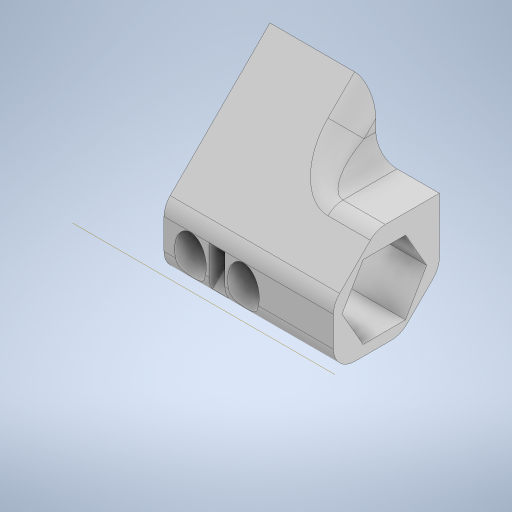
# Autodesk Inventor part: 2lickportv7
Saved by Autodesk Inventor 2024 (Build 280153000, 153)
## iProperties
Created: 2024-10-07
Part Number: 2lickportv7
Material: Generic
Document SubType Name: Modeling
Designer: xxred
Density: 1 g/cm^3
Appearance: Default
Author: xxred
Autodesk Inventor part; units mm, degrees
ref_plane "YZ Plane" through (0, 0, 0) normal (1, 0, 0) x (0, 1, 0)
ref_plane "XZ Plane" through (0, 0, 0) normal (0, 1, 0) x (-1, 0, 0)
ref_plane "XY Plane" through (0, 0, 0) normal (0, 0, 1) x (1, 0, 0)
sketch "Sketch2" plane through (0, 0, 0) normal (0, 1, 0) x (-1, 0, 0)
  line L0 (0, 0) -> (10, 0)
  line L1 (10, 0) -> (10, -10)
  line L2 (10, -10) -> (0, -10)
  line L3 (0, -10) -> (0, 0)
  dimension "d0" = 10
  dimension "d1" = 10
  constraints: 8 end point, 2 parallel, 1 horizontal, 1 perpendicular
  measures "d0" distance of L1.end L2.end
  measures "d1" distance of L0.end L1.end
extrude "Extrusion1" add sketch "Sketch2" along normal blind 20
ref_plane "Work Plane1" through (-10, 0, 0) normal (0, -0.7071068, 0.7071068) x (1, 0, 0)
sketch "Sketch3" plane through (-10, 0, 0) normal (0, -0.7071068, 0.7071068) x (1, 0, 0)
  circle A0 centre (2.5, 1.9025) radius 1.5
  circle A1 centre (7.5, 1.9025) radius 1.5
  line L0 (0, -7.0711) -> (0, 7.0711) projected
  line L1 (10, 0) -> (10, 14.1421) projected
  line L2 (0, 4.0177) -> (10, 4.0177)
  line L3 (10, 4.0177) -> (10, 14.1421)
  line L4 (10, 14.1421) -> (0, 14.1421)
  line L5 (0, 14.1421) -> (0, 4.0177)
  line L6 (2.5, 1.9025) -> (2.5, -0.2127)
  line L7 (2.5, 1.9025) -> (2.5, 4.0177)
  line L8 (4.25, 0.4025) -> (5.75, 0.4025)
  line L9 (5.75, 0.4025) -> (5.75, 3.4025)
  line L10 (5.75, 3.4025) -> (4.25, 3.4025)
  line L11 (4.25, 3.4025) -> (4.25, 0.4025)
  line L12 (7.5, 1.9025) -> (5.75, 1.9025)
  line L13 (4.25, 1.9025) -> (2.5, 1.9025)
  point P0 (10, 7.0711)
  dimension "d5" = 3
  dimension "d6" = 3
  dimension "d7" = 5
  dimension "d10" = 2.5
  dimension "d11" = 2.5
  dimension "d17" = 1.5
  dimension "d18" = 3
  constraints: 24 end point, 5 equal length, 3 perpendicular, 2 centre point, 2 collinear, 2 horizontal, 2 midpoint, 2 point on line, 1 vertical
  measures "d5" diameter of A0
  measures "d6" diameter of A1
  measures "d7" distance of L12.start L6.start
  measures "d10" distance from line of L0 L6.start
  measures "d11" distance from line of L1 L12.start
  measures "d17" distance of L9.end L10.end
  measures "d18" distance of L8.end L9.end
extrude "Extrusion2" cut sketch "Sketch3" against normal through all
sketch "Sketch4" plane through (0, 0, 0) normal (1, 0, 0) x (0, 0, -1)
  line L0 (8.8, 4.4641) -> (6.8, 1)
  line L1 (6.8, 1) -> (2.8, 1)
  line L2 (2.8, 1) -> (0.8, 4.4641)
  line L3 (0.8, 4.4641) -> (2.8, 7.9282)
  line L4 (2.8, 7.9282) -> (6.8, 7.9282)
  line L5 (6.8, 7.9282) -> (8.8, 4.4641)
  line L6 (0, 0) -> (10, 0) projected
  line L7 (10, 0) -> (10, 20) projected
  point P0 (4.8, 4.4641)
  point P1 (4.8, 1)
  point P2 (10, 15.6819)
  dimension "d12" = 4
  dimension "d13" = 1
  dimension "d14" = 1.2
  constraints: 12 end point, 1 midpoint, 1 parallel, 13 other
  measures "d12" distance of L3.end L4.end
  measures "d13" distance from line of point (4.8, 1) L6
  measures "d14" distance from line of L7 L0.start
sketch "Sketch5" plane through (0, 0, 0) normal (0, -1, 0) x (1, 0, 0)
  line L0 (0, 0) -> (0, -10) projected
  line L1 (0, 0) -> (6, 0)
  line L2 (6, 0) -> (6, -10)
  line L3 (6, -10) -> (0, -10)
  line L4 (0, -10) -> (0, 0)
  dimension "d19" = 6
  dimension "d20" = 10
  constraints: 8 end point, 2 parallel, 1 horizontal, 1 perpendicular
  measures "d19" distance of L2.end L3.end
  measures "d20" distance of L1.end L2.end
extrude "Extrusion4" add sketch "Sketch5" against normal blind 20
sketch "Sketch6" plane through (-10, 0, 0) normal (0, -0.7071068, 0.7071068) x (1, 0, 0)
  line L0 (0, 4.0177) -> (10, 4.0177) projected
  line L1 (10, 4.0177) -> (16.0958, 4.0177)
  line L2 (16.0958, 4.0177) -> (16.0958, 15.0177)
  line L3 (16.0958, 15.0177) -> (10, 15.0177)
  line L4 (10, 15.0177) -> (10, 4.0177)
  line L5 (0, -7.0711) -> (0, 4.0177) projected
  line L6 (16, -7.0711) -> (0, -7.0711) projected
  line L7 (0, -4.4836) -> (16, -4.4836)
  line L8 (16, -4.4836) -> (16, -7.0711)
  line L9 (16, -7.0711) -> (0, -7.0711)
  line L10 (0, -7.0711) -> (0, -4.4836)
  point P0 (10, 0)
  dimension "d32" = 11
  constraints: 16 end point, 4 parallel, 2 horizontal, 2 perpendicular, 1 point on line
  measures "d32" distance of L1.end L2.end
extrude "Extrusion5" cut sketch "Sketch6" against normal through all
extrude "Extrusion6" cut sketch "Sketch4" along normal blind 6
sketch "Sketch7" plane through (6, 0, 0) normal (1, 0, 0) x (0, 0, -1)
  line L0 (10, 15.6819) -> (0, 5.6819) projected
  line L1 (4.0697, 9.7516) -> (10, 9.7516)
  line L2 (10, 9.7516) -> (10, 15.6819)
  line L3 (10, 15.6819) -> (4.0697, 15.6819)
  line L4 (4.0697, 15.6819) -> (4.0697, 9.7516)
  point P0 (0, 0)
  constraints: 8 end point, 2 parallel, 1 horizontal, 1 perpendicular, 1 point on line
extrude "Extrusion7" cut sketch "Sketch7" against normal blind 6 contours L2 L1 L0
fillet "Fillet1" radius 2 1 edges at (0, 9.7516, -7.0348)
fillet "Fillet3" radius 2 7 edges at (0.5858, 10.3374, -4.6554) (4, 9.7516, -4.0697) (0, 13.7168, -8.0348) (-2, 5.6819, 0) (-2, 0, 0) (-2, 0, -6.3407) (-2, 3.6593, -10)
body "Solid1"
